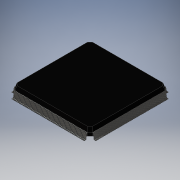
# Autodesk Inventor part: Cyclone3EPQ240
Saved by Autodesk Inventor 2016 (Build 200138000, 138)
## iProperties
Created: 2017-03-02
Part Number: Cyclone3EPQ240
Material: Generic
Document SubType Name: Modeling
Designer: jfixelle
Density: 1 g/cm^3
Appearance: Smooth - Black
Author: jfixelle
Autodesk Inventor part; units mm, degrees
ref_plane "XZ Plane" through (0, 0, 0) normal (0, 1, 0) x (-1, 0, 0)
ref_plane "XY Plane" through (0, 0, 0) normal (0, 0, 1) x (1, 0, 0)
sketch "Sketch1" plane through (0, 0, 0) normal (0, 1, 0) x (-1, 0, 0)
  line L0 (16, 16) -> (-16, 16)
  line L1 (-16, 16) -> (-16, -16)
  line L2 (-16, -16) -> (16, -16)
  line L3 (16, -16) -> (16, 16)
  point P0 (0, 0)
  dimension "d0" = 32
  dimension "d1" = 32
  dimension "d2" = 16
  dimension "d3" = 16
  constraints: 8 end point, 2 parallel, 1 horizontal, 1 perpendicular
  measures "d0" distance of L2.end L0.start
  measures "d1" distance of L1.end L2.end
  measures "d2" distance from line of point (0, 0) L3
  measures "d3" distance from line of point (0, 0) L2
extrude "Extrusion1" add sketch "Sketch1" along normal blind 3.55
chamfer "Chamfer1" distance 1.775 angle 15 1 edges at (0, 0, 16) measured on face at (-5.3333, 1.1833, 16)
chamfer "Chamfer2" distance 1.775 angle 15 1 edges at (16, 0, -0.2378) measured on face at (16, 2.3667, 5.1748)
chamfer "Chamfer3" distance 1.775 angle 15 1 edges at (-0.2378, 0, -16) measured on face at (5.1748, 2.3667, -16)
chamfer "Chamfer4" distance 1.775 angle 15 1 edges at (-16, 0, 0) measured on face at (-16, 2.3667, 5.1748)
chamfer "Chamfer5" distance 1.775 angle 15 1 edges at (-16, 3.55, 0) measured on face at (-16, 2.3667, -5.3333)
chamfer "Chamfer6" distance 1.775 angle 15 1 edges at (0.2378, 3.55, 16) measured on face at (-5.1748, 2.3667, 16)
chamfer "Chamfer7" distance 1.775 angle 15 1 edges at (0.2378, 3.55, -16) measured on face at (-5.1748, 2.3667, -16)
chamfer "Chamfer8" distance 1.775 angle 15 1 edges at (16, 3.55, 0) measured on face at (16, 2.3667, 5.1748)
chamfer "Chamfer9" distance 1 angle 45 2 edges at (-15.7622, 0.8875, 15.7622) (-15.7622, 2.6625, 15.7622)
chamfer "Chamfer10" distance 1 angle 45 6 edges at (-15.7622, 0.8875, -15.7622) (-15.7622, 2.6625, -15.7622) (15.7622, 0.8875, 15.7622) (15.7622, 2.6625, 15.7622) (15.7622, 0.8875, -15.7622) (15.7622, 2.6625, -15.7622)
ref_plane "Work Plane1" through (0.25, 0, 0) normal (1, 0, 0) x (0, 1, 0)
sketch "Sketch2" plane through (0.25, 0, 0) normal (1, 0, 0) x (0, 1, 0)
  line L0 (1.8567, 14.7365) -> (1.8567, 16.3287)
  line L1 (1.8567, 16.3287) -> (-0.35, 16.7178)
  line L2 (-0.35, 16.7178) -> (-0.35, 17.3)
  line L3 (-0.35, 17.3) -> (-0.55, 17.3)
  line L4 (-0.55, 17.3) -> (-0.55, 16.55)
  line L5 (-0.55, 16.55) -> (1.6567, 16.1609)
  line L6 (1.6567, 16.1609) -> (1.6567, 14.7365)
  line L7 (1.6567, 14.7365) -> (1.8567, 14.7365)
  line L8 (0, 0) -> (-0.0235, 0)
  line L9 (0, 15.5244) -> (0, 14.4914) projected
  dimension "d37" = 17.3
  dimension "d38" = 0.75
  dimension "d39" = 0.55
  dimension "d40" = 0.2
  dimension "d41" = 0.2
  dimension "d42" = 80
  dimension "d43" = 0.2
  constraints: 18 end point, 3 parallel, 3 perpendicular, 1 horizontal, 1 vertical
  measures "d37" distance between parallel lines of L3 L8
  measures "d38" distance of L3.end L4.end
  measures "d39" distance between parallel lines of L9 L4
  measures "d40" distance of L2.end L3.end
  measures "d41" distance between parallel lines of L6 L0
  measures "d42" angle of L2 L1
  measures "d43" distance between parallel lines of L5 L1
extrude "Extrusion2" add sketch "Sketch2" along normal mid plane 0.27
pattern_linear "Rectangular Pattern1" count 60 spacing 0.5 along (-1, 0, 0) of "Extrusion2" first direction both ways yes
pattern_circular "Circular Pattern1" count 4 over 360 about axis through (0, -10, 0) along (0, 1, 0) of "Extrusion2", "Rectangular Pattern1"
body "Solid1"
